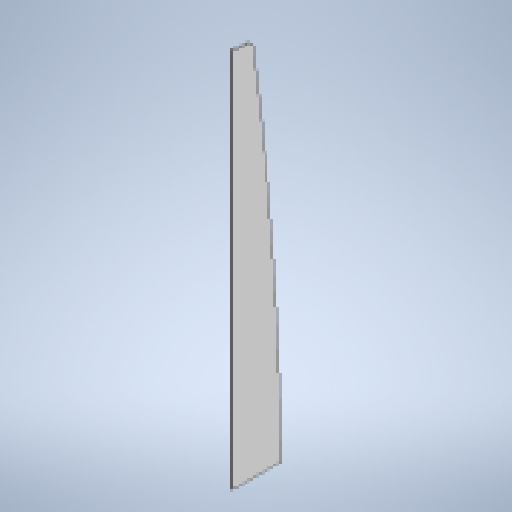
# Autodesk Inventor part: MSC 079 top pillar
Saved by Autodesk Inventor 2025 (Build 290162010, 162A)
## iProperties
Created: 2024-08-30
Part Number: MSC 079 top pillar
Material: Stainless Steel
Document SubType Name: Sheet Metal
Designer: pokla
Density: 8 g/cm^3
Sheet Metal Rule: AISI304 3mm Die 32
Appearance: Default
Author: pokla
Autodesk Inventor part; units mm, degrees
ref_plane "YZ Plane" through (0, 0, 0) normal (1, 0, 0) x (0, 1, 0)
ref_plane "XZ Plane" through (0, 0, 0) normal (0, 1, 0) x (-1, 0, 0)
ref_plane "XY Plane" through (0, 0, 0) normal (0, 0, 1) x (1, 0, 0)
sketch "Sketch1" plane through (0, 0, 0) normal (1, 0, 0) x (0, 1, 0)
  line L0 (34.288, 751) -> (0, 751)
  line L1 (0, 751) -> (0, -751)
  line L2 (0, -751) -> (34.288, -751)
  arc A0 (34.288, -751) -> (34.288, 751) centre (-5565.578, 0) ccw
  line L3 (0, 751) -> (34.6778, 748.088)
  line L4 (0, -751) -> (34.6778, -748.088)
  line L5 (0, 97) -> (83.5893, 97)
  point P0 (0, 0)
  point P1 (0, 0)
  dimension "d1" = 1502
  dimension "d2" = 34.288
  dimension "d3" = 5650
  dimension "d7" = 85.2
  dimension "d8" = 85.2
  dimension "d19" = 654
  measures "d1" distance of L0.end L1.end
  measures "d2" distance of L0.start L0.end
  measures "d3" radius of A0
  measures "d7" angle of L1 L3
  measures "d8" angle of L1 L4
  measures "d19" distance of L5.start L0.end
extrude "Plate1" add sketch "Sketch1" against normal blind 3.048 contours L3 A0 L5 L1
fillet "Corner Round3" radius 10 1 edges at (-1.524, 34.6778, 748.088)
sketch "Sketch4" plane through (0, 0, 0) normal (1, 0, 0) x (0, 0, -1)
  circle A0 centre (-728, 10) radius 3.5
  line L0 (-751, 0) -> (-97, 0) projected
  point P0 (0, 0)
  dimension "d23" = 7
  dimension "d24" = 631
  dimension "d25" = 10
  constraints: 1 centre point
  measures "d23" diameter of A0
  measures "d24" horizontal distance of L0.end A0.centre
  measures "d25" distance from line of L0 A0.centre
extrude "Extrusion1" cut sketch "Sketch4" against normal through all
pattern_linear "Rectangular Pattern2" count 9 spacing 63 along (0, 0, -1) of "Extrusion1"
equation "\"BendReliefWidth\" = Thickness"
equation "\"BendReliefDepth\" = 0.5 * Thickness"
equation "\"CornerReliefSize\" = 4 * Thickness"
equation "\"MinimumRemnant\" = 2 * Thickness"
equation "\"TransitionRadius\" = BendRadius"
equation "\"JacobiRadiusSize\" = BendRadius"
equation "\"GapSize\" = Thickness"
equation "\"BendRadius\" = Thickness"
body "Solid1"
